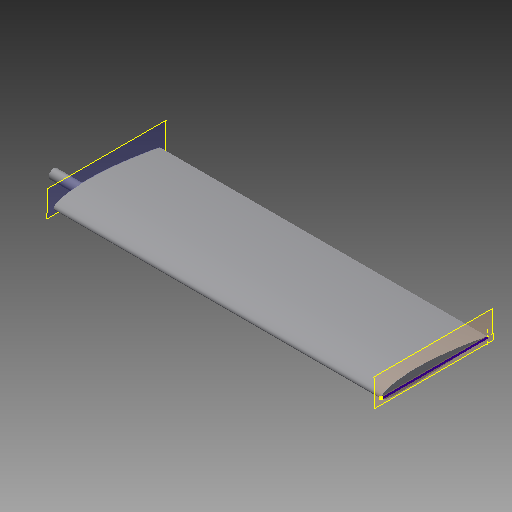
# Autodesk Inventor part: Generic Wing 1
Saved by Autodesk Inventor 2018 (Build 220112000, 112)
## iProperties
Created: 2018-07-21
Part Number: Generic Wing 1
Material: Generic
Document SubType Name: Modeling
Designer: Michael Gunderman
Density: 0.0908399 g/cm^3
Appearance: Default
Mass: 500 g
Surface Area: 5034.56 cm^2
Volume: 5504.19 cm^3
Author: Michael Gunderman
Autodesk Inventor part; units mm, degrees
ref_plane "YZ Plane" through (0, 0, 0) normal (1, 0, 0) x (0, 1, 0)
ref_plane "XZ Plane" through (0, 0, 0) normal (0, 1, 0) x (-1, 0, 0)
ref_plane "XY Plane" through (0, 0, 0) normal (0, 0, 1) x (1, 0, 0)
sketch "Sketch1" plane through (0, 0, 0) normal (1, 0, 0) x (0, 1, 0)
  spline S0 degree 4 poles (0.3627, -279) (2.947, -266.0312) (4.0152, -261.9095) (10.1054, -227.3355) (14.5376, -195.2827) (17.9783, -167.5351) (20.2676, -139.4009) (21.9893, -115.461) (22.209, -84.8272) (21.647, -71.9934) (20.3849, -55.8209) (18.902, -43.6327) (16.1047, -28.5338) (14.0079, -21.7205) (12.2118, -14.8155) (8.0674, -6.4124) (7.079, -4.2379) (-0.1183, 2.7681) (-5.3228, -4.1519) (-6.264, -6.518) (-8.9097, -14.9218) (-9.7575, -21.7589) (-10.6673, -28.6215) (-11.659, -43.7118) (-11.86, -55.8663) (-11.8135, -72.0242) (-11.4845, -84.8406) (-10.5616, -115.4432) (-9.3798, -139.3719) (-7.7193, -167.4754) (-5.969, -195.2313) (-3.9919, -227.2327) (-1.5095, -261.8448) (-1.3026, -266.0273) (-0.3627, -279) knots 0 0 0 0 0 0.079164 0.11599 0.155667 0.195283 0.234849 0.271492 0.305234 0.336106 0.36415 0.390233 0.414389 0.436709 0.455812 0.474816 0.493245 0.510185 0.528336 0.546539 0.565204 0.587171 0.611081 0.636996 0.664941 0.695772 0.7295 0.76613 0.80566 0.845199 0.884743 0.921395 1 1 1 1 1
  line L0 (0.3627, -279) -> (0, -279.3915)
  line L1 (0, -279.3915) -> (-0.3627, -279)
  point P0 (0, 0)
  point P1 (3.1806, -265.05)
  point P2 (5.8032, -251.1)
  point P3 (10.4625, -223.2)
  point P4 (14.4522, -195.3)
  point P5 (17.7444, -167.4)
  point P6 (20.1996, -139.5)
  point P7 (21.762, -111.6)
  point P8 (21.9852, -83.7)
  point P9 (21.3993, -69.75)
  point P10 (20.2554, -55.8)
  point P11 (18.4419, -41.85)
  point P12 (15.7077, -27.9)
  point P13 (13.8384, -20.925)
  point P14 (11.5227, -13.95)
  point P15 (8.3421, -6.975)
  point P16 (5.9985, -3.4875)
  point P17 (0, 0)
  point P18 (-4.6035, -3.4875)
  point P19 (-6.3333, -6.975)
  point P20 (-8.3979, -13.95)
  point P21 (-9.6534, -20.925)
  point P22 (-10.4625, -27.9)
  point P23 (-11.439, -41.85)
  point P24 (-11.8017, -55.8)
  point P25 (-11.7738, -69.75)
  point P26 (-11.4948, -83.7)
  point P27 (-10.602, -111.6)
  point P28 (-9.3186, -139.5)
  point P29 (-7.7004, -167.4)
  point P30 (-5.9706, -195.3)
  point P31 (-4.185, -223.2)
  point P32 (-2.2878, -251.1)
  point P33 (-1.3392, -265.05)
  point P34 (8.3421, -6.975)
  constraints: 4 end point, 1 coincident, 35 other
extrude "Extrusion1" add sketch "Sketch1" along normal blind 860
sketch "Sketch2" plane through (860, 0, 0) normal (1, 0, 0) x (0, 0, -1)
  line L0 (1.5803, -0.3627) -> (279, -0.3627)
  point P0 (0, 0)
  constraints: 2 end point, 1 horizontal
ref_plane "Work Plane1" through (860, -0.3627, -1.5803) normal (0.9993908, 0.0348995, 0) x (0, 0, -1)
ref_plane "Work Plane2" through (430, 0, 0) normal (1, 0, 0) x (0, 0, -1)
pattern_of_nothing "Mirror1"
sketch "Sketch3" plane through (0, 0, 0) normal (-1, 0, 0) x (0, 0, 1)
  line L0 (-74.6615, 5.1053) -> (0, 0) construction
  circle A0 centre (-74.6615, 5.1053) radius 12.7
  dimension "d3" = 25.4
  constraints: 2 end point, 1 centre point, 1 coincident
  measures "d3" diameter of A0
extrude "Extrusion2" add sketch "Sketch3" along normal blind 74
ref_plane "Work Plane3" through (0, -0.3627, -1.5803) normal (0.9993908, -0.0348995, 0) x (0, 0, -1)
body "Solid1"
